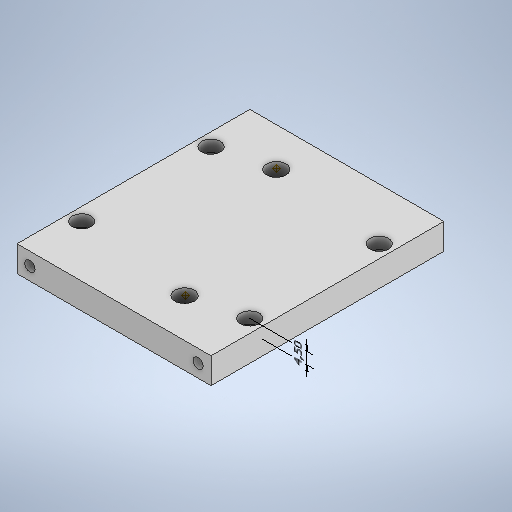
# Autodesk Inventor part: Rb PEEK - Arriba
Saved by Autodesk Inventor 2025.3 (Build 293356000, 356)
## iProperties
Created: 2025-05-09
Part Number: Rb PEEK - Arriba
Material: Generic
Document SubType Name: Modeling
Designer: E. Moreno
Density: 1 g/cm^3
Appearance: Default
Title: Rb PEEK - Arriba
Author: E. Moreno
Autodesk Inventor part; units mm, degrees
ref_plane "YZ Plane" through (0, 0, 0) normal (1, 0, 0) x (0, 1, 0)
ref_plane "XZ Plane" through (0, 0, 0) normal (0, 1, 0) x (-1, 0, 0)
ref_plane "XY Plane" through (0, 0, 0) normal (0, 0, 1) x (1, 0, 0)
sketch "Sketch1" plane through (0, 0, 0) normal (0, 1, 0) x (-1, 0, 0)
  line L0 (-37.5, 45) -> (37.5, 45)
  line L1 (37.5, 45) -> (37.5, -45)
  line L2 (37.5, -45) -> (-37.5, -45)
  line L3 (-37.5, -45) -> (-37.5, 45)
  line L4 (-37.5, 45) -> (37.5, -45) construction
  line L5 (37.5, 45) -> (-37.5, -45) construction
  point P0 (0, 0)
  dimension "d0" = 75
  dimension "d1" = 90
  constraints: 12 end point, 2 midpoint, 2 parallel, 1 horizontal, 1 perpendicular
  measures "d0" distance of L1.end L2.end
  measures "d1" distance of L0.end L1.end
extrude "Extrusion1" add sketch "Sketch1" along normal blind 10
sketch "Sketch2" plane through (0, 10, 0) normal (0, 1, 0) x (1, 0, 0)
  line L0 (-37.5, -45) -> (37.5, -45) projected
  line L1 (37.5, -45) -> (37.5, -25)
  line L2 (37.5, -45) -> (37.5, 45) projected
  line L3 (37.5, -25) -> (32.5, -25)
  circle A0 centre (32.5, -25) radius 2
  line L4 (0, 0) -> (37.5, 0)
  line L5 (-37.5, 45) -> (37.5, 45)
  line L6 (37.5, 45) -> (37.5, 25)
  line L7 (37.5, 45) -> (37.5, -45)
  line L8 (37.5, 25) -> (32.5, 25)
  circle A1 centre (32.5, 25) radius 2
  line L9 (0, -45) -> (0, 45)
  line L10 (-37.5, -45) -> (-37.5, -25)
  line L11 (-37.5, -45) -> (-37.5, 45)
  line L12 (-37.5, -25) -> (-32.5, -25)
  circle A2 centre (-32.5, -25) radius 2
  line L13 (-37.5, 45) -> (-37.5, 25)
  line L14 (-37.5, 45) -> (-37.5, -45)
  line L15 (-37.5, 25) -> (-32.5, 25)
  circle A3 centre (-32.5, 25) radius 2
  point P0 (-37.5, 0)
  dimension "d4" = 20
  dimension "d5" = 5
  dimension "d6" = 4
  constraints: 28 end point, 17 symmetric about line, 4 centre point, 4 coincident, 4 point on line, 3 midpoint, 1 horizontal, 3 other
  measures "d4" distance of L0.end L1.end
  measures "d5" distance of L1.end L3.end
  measures "d6" diameter of A0
extrude "Extrusion2" cut sketch "Sketch2" against normal blind 10 contours A0 | A1 | A2 | A3
sketch "Sketch3" plane through (0, 10, 0) normal (0, 1, 0) x (1, 0, 0)
  circle A0 centre (32.5, -25) radius 3.61
  circle A1 centre (32.5, -25) radius 2 projected
  line L0 (0, 0) -> (29.9913, 0)
  line L1 (-37.5, -45) -> (37.5, -45) projected
  line L2 (0, -45) -> (0, 45)
  circle A2 centre (32.5, -25) radius 2
  circle A3 centre (32.5, 25) radius 3.61
  circle A4 centre (32.5, 25) radius 2
  circle A5 centre (32.5, 25) radius 2
  circle A6 centre (-32.5, -25) radius 3.61
  circle A7 centre (-32.5, -25) radius 2
  circle A8 centre (-32.5, -25) radius 2
  circle A9 centre (-32.5, 25) radius 3.61
  circle A10 centre (-32.5, 25) radius 2
  circle A11 centre (-32.5, 25) radius 2
  point P0 (-29.9913, 0)
  dimension "d11" = 7.22
  dimension "d14" = 4
  constraints: 11 centre point, 10 symmetric about line, 4 end point, 2 concentric, 1 horizontal, 1 midpoint, 9 other
  measures "d11" diameter of A0
  measures "d14" diameter of A2
extrude "Extrusion3" cut sketch "Sketch3" against normal blind 4.5
sketch "Sketch4" plane through (0, 10, 0) normal (0, 1, 0) x (1, 0, 0)
  line L0 (-37.5, -45) -> (37.5, -45) projected
  line L1 (37.5, -45) -> (12.25, -45)
  line L2 (12.25, -45) -> (12.25, -30)
  circle A0 centre (12.25, -30) radius 3.75
  line L3 (37.5, 45) -> (-37.5, 45) projected
  line L4 (-37.5, 45) -> (-12.25, 45)
  line L5 (-12.25, 45) -> (-12.25, 30)
  circle A1 centre (-12.25, 30) radius 3.75
  point P0 (0, 0)
  dimension "d17" = 25.25
  dimension "d18" = 15
  dimension "d19" = 7.5
  dimension "d22" = 25.25
  dimension "d23" = 15
  dimension "d24" = 7.5
  constraints: 8 end point, 2 centre point, 2 coincident, 2 point on line, 1 perpendicular, 1 vertical
  measures "d17" distance of L0.end L1.end
  measures "d18" distance of L1.end L2.end
  measures "d19" diameter of A0
  measures "d22" distance of L3.end L4.end
  measures "d23" distance of L4.end L5.end
  measures "d24" diameter of A1
extrude "Extrusion5" cut sketch "Sketch4" against normal blind 10
sketch "Sketch7" plane through (0, 10, 0) normal (0, 1, 0) x (1, 0, 0)
  circle A0 centre (-12.25, 30) radius 3.75 projected
sketch "Sketch8" plane through (0, 10, 0) normal (0, 1, 0) x (1, 0, 0)
  circle A0 centre (12.25, -30) radius 3.75 projected
sketch "Sketch9" plane through (-37.5, 0, 45) normal (0, 0, 1) x (1, 0, 0)
  line L0 (0, 0) -> (0, 10) projected
  line L1 (0, 5) -> (5, 5)
  circle A0 centre (5, 5) radius 2
  line L2 (75, 0) -> (75, 10) projected
  line L3 (75, 5) -> (70, 5)
  circle A1 centre (70, 5) radius 2
  point P0 (37.5, 0)
  dimension "d28" = 5
  dimension "d29" = 4
  dimension "d30" = 5
  dimension "d31" = 4
  constraints: 4 end point, 2 centre point, 2 coincident, 2 horizontal, 2 midpoint
  measures "d28" distance of L1.start L1.end
  measures "d29" diameter of A0
  measures "d30" distance of L3.start L3.end
  measures "d31" diameter of A1
sketch "Sketch10" plane through (37.5, 0, -45) normal (0, 0, -1) x (-1, 0, 0)
  line L0 (0, 0) -> (0, 10) projected
  line L1 (0, 5) -> (5, 5)
  line L2 (75, 0) -> (75, 10) projected
  line L3 (75, 5) -> (70, 5)
  circle A0 centre (5, 5) radius 2
  circle A1 centre (70, 5) radius 2
  point P0 (37.5, 0)
  dimension "d32" = 5
  dimension "d33" = 5
  dimension "d34" = 4
  dimension "d35" = 4
  constraints: 4 end point, 2 centre point, 2 coincident, 2 horizontal, 2 midpoint
  measures "d32" distance of L1.start L1.end
  measures "d33" distance of L3.start L3.end
  measures "d34" diameter of A0
  measures "d35" diameter of A1
extrude "Extrusion6" cut sketch "Sketch10" against normal blind 15
extrude "Extrusion7" cut sketch "Sketch9" against normal blind 15
thread "Thread1" size "M4x0.7" class "6H" standard "ANSI Metric M Profile" full length
thread "Thread2" size "M4x0.7" class "6H" standard "ANSI Metric M Profile" full length
thread "Thread3" size "M4x0.7" class "6H" standard "ANSI Metric M Profile" full length
thread "Thread4" size "M4x0.7" class "6H" standard "ANSI Metric M Profile" full length
body "Solid1"
